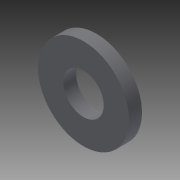
# Autodesk Inventor part: 0.56250.0800000000000001-rod_part
Saved by Autodesk Inventor 2014 (Build 180170000, 170)
## iProperties
Created: 2014-01-19
Part Number: 0.56250.0800000000000001-rod_part
Material: Generic
Catalog Web Link: www.cadenas.de
Description: FO1-Rod Part-Bimba FLAT-1
Vendor: BIMBA
Document SubType Name: Standard Catalog Part
Designer: Andrew Toennies
Manufacturer: BIMBA
Density: 1 g/cm^3
Appearance: RGB(180.00000447034725,180.00000447034725,180.00000447034725)
Category: PARTsolutions
Company: BIMBA
Title: 0.56250.0800000000000001-rod_part
Author: Cadenas PARTsolutions
Comments: Bimba FLAT-1
PSOL_IDENT_0: {$CADENAS_DATA\23d-libs\bimba\bimba\bimba_imperial\bimba_full_line\flat_cylinders\fo1\fo1_rod_part.p
PSOL_IDENT_1: rj},215 {VTYP=3D},{NB=0.56250.0800000000000001-rod_part},{LINA=0.56250.0800000000000001-rod_part},{N
PSOL_IDENT_2: N=FO1-Rod Part},{DATE=08.03.2011 12:37:02},{GEOMDATE=04.03.2011 10:19:00},{VERSION=},{LINEID=10},{LI
PSOL_IDENT_3: NESUBID=-1},{WBVAR=L}  {NB=0.56250.0800000000000001-rod_part},{LINA=0.56250.0800000000000001-rod_par
PSOL_IDENT_4: t},{KT=DUMMY},{PN=0.56250.0800000000000001-rod_part},{BORE=0.56250000},{L=0.0800000000000001},{TDIN=
PSOL_IDENT_5: 0.56200000},{F=0.25000000}
CNS_NN: FO1-Rod Part
CNS_NT: Bimba FLAT-1
CNS_NB: 0.56250.0800000000000001-rod_part
CNS_NBSYN: $PN.
CNS_LINA: 0.56250.0800000000000001-rod_part
CNS_PN: 0.56250.0800000000000001-rod_part
CNS_BORE: 0.56250000
CNS_L: 0.0800000000000001
CNS_TDIN: 0.56200000
CNS_F: 0.25000000
SUPPLIER: BIMBA
ARTICLENO: 0.56250.0800000000000001-rod_part
BOMINFO: 0.56250.0800000000000001-rod_part
CREATOR: CADENAS GmbH
Autodesk Inventor part; units mm, degrees
ref_plane "YZ Plane" through (0, 0, 0) normal (1, 0, 0) x (0, 1, 0)
ref_plane "XZ Plane" through (0, 0, 0) normal (0, 1, 0) x (-1, 0, 0)
ref_plane "XY Plane" through (0, 0, 0) normal (0, 0, 1) x (1, 0, 0)
sketch "Sketch_1" plane through (0, 0, 0) normal (1, 0, 0) x (0, 1, 0)
  line L0 (0, -2.032) -> (0, 0)
  line L1 (7.1374, 0) -> (3.175, 0)
  line L2 (3.175, 0) -> (3.175, -2.032)
  line L3 (3.175, -2.032) -> (7.1374, -2.032)
  line L4 (7.1374, -2.032) -> (7.1374, 0)
  constraints: 10 end point
revolve "Revolution1" add sketch "Sketch_1" angle 360 about axis through (0, 0, -2.032) along (0, 0, -1)
ref_plane "part_to_rod_XY" through (0, 0, 0) normal (0, 0, 1) x (1, 0, 0)
ref_plane "part_to_rod_YZ" through (0, 0, 0) normal (1, 0, 0) x (0, 1, 0)
ref_plane "part_to_rod_ZX" through (0, 0, 0) normal (0, 1, 0) x (0, 0, 1)
body "Solid1"
